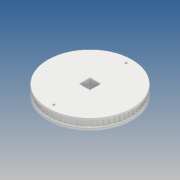
# Autodesk Inventor part: Poleas de transmision 60Dientes (ZR timing belts)
Saved by Autodesk Inventor 2020 (Build 240168000, 168)
## iProperties
Part Number: Poleas de transmision 60Dientes (ZR timing belts)
Material: Genérico
Document SubType Name: Modeling
Designer: FABLAB
Density: 1 g/cm^3
Appearance: Blanco
Description: Acrílico corte laser CNC
Author: FABLAB
Autodesk Inventor part; units mm, degrees
ref_plane "YZ Plane" through (0, 0, 0) normal (1, 0, 0) x (0, 1, 0)
ref_plane "XZ Plane" through (0, 0, 0) normal (0, 1, 0) x (-1, 0, 0)
ref_plane "XY Plane" through (0, 0, 0) normal (0, 0, 1) x (1, 0, 0)
sketch "Boceto1" plane through (0, 0, 0) normal (0, 0, 1) x (1, 0, 0)
  line L0 (8, -8) -> (-8, -8) projected
  line L1 (-8, -8) -> (-8, 8) projected
  line L2 (-8, 8) -> (8, 8) projected
  line L3 (8, 8) -> (8, -8) projected
  circle A0 centre (0, 0) radius 15 construction
  circle A1 centre (0, 0) radius 60
  circle A2 centre (0, 0) radius 55 construction
  circle A3 centre (0, 55) radius 1.5
  circle A4 centre (0, -55) radius 1.5
  circle A5 centre (0, 0) radius 61.2874 construction
  line L4 (-1.5392, 59.9803) -> (1.5392, 59.9803)
  line L5 (1.5392, 59.9803) -> (0.933, 61.2803)
  line L6 (0.933, 61.2803) -> (-0.933, 61.2803)
  line L7 (-0.933, 61.2803) -> (-1.5392, 59.9803)
  line L8 (0, 59.9803) -> (0, 0) construction
  line L9 (0, 0) -> (2.5392, 59.9462) construction
  line L10 (0, 0) -> (-2.5392, 59.9462) construction
  arc A6 (-2.5392, 59.9462) -> (2.5392, 59.9462) centre (0, 119.8925) ccw construction
  line L11 (1.5392, 59.9803) -> (1.5392, 62.0856) construction
  line L12 (-7.3335, 60.847) -> (-7.8005, 59.4908)
  line L13 (-5.4776, 61.0421) -> (-7.3335, 60.847)
  line L14 (-4.7388, 59.8126) -> (-5.4776, 61.0421)
  line L15 (-13.6535, 59.7471) -> (-13.9762, 58.3495)
  line L16 (-11.8282, 60.1351) -> (-13.6535, 59.7471)
  line L17 (-10.965, 58.9896) -> (-11.8282, 60.1351)
  line L18 (-19.824, 57.9927) -> (-19.9988, 56.569)
  line L19 (-18.0493, 58.5693) -> (-19.824, 57.9927)
  line L20 (-17.071, 57.5203) -> (-18.0493, 58.5693)
  line L21 (-25.7773, 55.6028) -> (-25.8023, 54.1686)
  line L22 (-24.0725, 56.3618) -> (-25.7773, 55.6028)
  line L23 (-22.99, 55.4208) -> (-24.0725, 56.3618)
  line L24 (-31.4482, 52.6037) -> (-31.3231, 51.1748)
  line L25 (-29.8321, 53.5368) -> (-31.4482, 52.6037)
  line L26 (-28.6571, 52.714) -> (-29.8321, 53.5368)
  line L27 (-36.7745, 49.0283) -> (-36.5008, 47.6203)
  line L28 (-35.2648, 50.1252) -> (-36.7745, 49.0283)
  line L29 (-34.0102, 49.4298) -> (-35.2648, 50.1252)
  line L30 (-41.6979, 44.9158) -> (-41.2785, 43.5441)
  line L31 (-40.3111, 46.1644) -> (-41.6979, 44.9158)
  line L32 (-38.9907, 45.604) -> (-40.3111, 46.1644)
  line L33 (-46.1644, 40.3111) -> (-45.604, 38.9907)
  line L34 (-44.9158, 41.6979) -> (-46.1644, 40.3111)
  line L35 (-43.5441, 41.2785) -> (-44.9158, 41.6979)
  line L36 (-50.1252, 35.2648) -> (-49.4298, 34.0102)
  line L37 (-49.0283, 36.7745) -> (-50.1252, 35.2648)
  line L38 (-47.6203, 36.5008) -> (-49.0283, 36.7745)
  line L39 (-53.5368, 29.8321) -> (-52.714, 28.6571)
  line L40 (-52.6037, 31.4482) -> (-53.5368, 29.8321)
  line L41 (-51.1748, 31.3231) -> (-52.6037, 31.4482)
  line L42 (-56.3618, 24.0725) -> (-55.4208, 22.99)
  line L43 (-55.6028, 25.7773) -> (-56.3618, 24.0725)
  line L44 (-54.1686, 25.8023) -> (-55.6028, 25.7773)
  line L45 (-58.5693, 18.0493) -> (-57.5203, 17.071)
  line L46 (-57.9927, 19.824) -> (-58.5693, 18.0493)
  line L47 (-56.569, 19.9988) -> (-57.9927, 19.824)
  line L48 (-60.1351, 11.8282) -> (-58.9896, 10.965)
  line L49 (-59.7471, 13.6535) -> (-60.1351, 11.8282)
  line L50 (-58.3495, 13.9762) -> (-59.7471, 13.6535)
  line L51 (-61.0421, 5.4776) -> (-59.8126, 4.7388)
  line L52 (-60.847, 7.3335) -> (-61.0421, 5.4776)
  line L53 (-59.4908, 7.8005) -> (-60.847, 7.3335)
  line L54 (-61.2803, -0.933) -> (-59.9803, -1.5392)
  line L55 (-61.2803, 0.933) -> (-61.2803, -0.933)
  line L56 (-59.9803, 1.5392) -> (-61.2803, 0.933)
  line L57 (-60.847, -7.3335) -> (-59.4908, -7.8005)
  line L58 (-61.0421, -5.4776) -> (-60.847, -7.3335)
  line L59 (-59.8126, -4.7388) -> (-61.0421, -5.4776)
  line L60 (-59.7471, -13.6535) -> (-58.3495, -13.9762)
  line L61 (-60.1351, -11.8282) -> (-59.7471, -13.6535)
  line L62 (-58.9896, -10.965) -> (-60.1351, -11.8282)
  line L63 (-57.9927, -19.824) -> (-56.569, -19.9988)
  line L64 (-58.5693, -18.0493) -> (-57.9927, -19.824)
  line L65 (-57.5203, -17.071) -> (-58.5693, -18.0493)
  line L66 (-55.6028, -25.7773) -> (-54.1686, -25.8023)
  line L67 (-56.3618, -24.0725) -> (-55.6028, -25.7773)
  line L68 (-55.4208, -22.99) -> (-56.3618, -24.0725)
  line L69 (-52.6037, -31.4482) -> (-51.1748, -31.3231)
  line L70 (-53.5368, -29.8321) -> (-52.6037, -31.4482)
  line L71 (-52.714, -28.6571) -> (-53.5368, -29.8321)
  line L72 (-49.0283, -36.7745) -> (-47.6203, -36.5008)
  line L73 (-50.1252, -35.2648) -> (-49.0283, -36.7745)
  line L74 (-49.4298, -34.0102) -> (-50.1252, -35.2648)
  line L75 (-44.9158, -41.6979) -> (-43.5441, -41.2785)
  line L76 (-46.1644, -40.3111) -> (-44.9158, -41.6979)
  line L77 (-45.604, -38.9907) -> (-46.1644, -40.3111)
  line L78 (-40.3111, -46.1644) -> (-38.9907, -45.604)
  line L79 (-41.6979, -44.9158) -> (-40.3111, -46.1644)
  line L80 (-41.2785, -43.5441) -> (-41.6979, -44.9158)
  line L81 (-35.2648, -50.1252) -> (-34.0102, -49.4298)
  line L82 (-36.7745, -49.0283) -> (-35.2648, -50.1252)
  line L83 (-36.5008, -47.6203) -> (-36.7745, -49.0283)
  line L84 (-29.8321, -53.5368) -> (-28.6571, -52.714)
  line L85 (-31.4482, -52.6037) -> (-29.8321, -53.5368)
  line L86 (-31.3231, -51.1748) -> (-31.4482, -52.6037)
  line L87 (-24.0725, -56.3618) -> (-22.99, -55.4208)
  line L88 (-25.7773, -55.6028) -> (-24.0725, -56.3618)
  line L89 (-25.8023, -54.1686) -> (-25.7773, -55.6028)
  line L90 (-18.0493, -58.5693) -> (-17.071, -57.5203)
  line L91 (-19.824, -57.9927) -> (-18.0493, -58.5693)
  line L92 (-19.9988, -56.569) -> (-19.824, -57.9927)
  line L93 (-11.8282, -60.1351) -> (-10.965, -58.9896)
  line L94 (-13.6535, -59.7471) -> (-11.8282, -60.1351)
  line L95 (-13.9762, -58.3495) -> (-13.6535, -59.7471)
  line L96 (-5.4776, -61.0421) -> (-4.7388, -59.8126)
  line L97 (-7.3335, -60.847) -> (-5.4776, -61.0421)
  line L98 (-7.8005, -59.4908) -> (-7.3335, -60.847)
  line L99 (0.933, -61.2803) -> (1.5392, -59.9803)
  line L100 (-0.933, -61.2803) -> (0.933, -61.2803)
  line L101 (-1.5392, -59.9803) -> (-0.933, -61.2803)
  line L102 (7.3335, -60.847) -> (7.8005, -59.4908)
  line L103 (5.4776, -61.0421) -> (7.3335, -60.847)
  line L104 (4.7388, -59.8126) -> (5.4776, -61.0421)
  line L105 (13.6535, -59.7471) -> (13.9762, -58.3495)
  line L106 (11.8282, -60.1351) -> (13.6535, -59.7471)
  line L107 (10.965, -58.9896) -> (11.8282, -60.1351)
  line L108 (19.824, -57.9927) -> (19.9988, -56.569)
  line L109 (18.0493, -58.5693) -> (19.824, -57.9927)
  line L110 (17.071, -57.5203) -> (18.0493, -58.5693)
  line L111 (25.7773, -55.6028) -> (25.8023, -54.1686)
  line L112 (24.0725, -56.3618) -> (25.7773, -55.6028)
  line L113 (22.99, -55.4208) -> (24.0725, -56.3618)
  line L114 (31.4482, -52.6037) -> (31.3231, -51.1748)
  line L115 (29.8321, -53.5368) -> (31.4482, -52.6037)
  line L116 (28.6571, -52.714) -> (29.8321, -53.5368)
  line L117 (36.7745, -49.0283) -> (36.5008, -47.6203)
  line L118 (35.2648, -50.1252) -> (36.7745, -49.0283)
  line L119 (34.0102, -49.4298) -> (35.2648, -50.1252)
  line L120 (41.6979, -44.9158) -> (41.2785, -43.5441)
  line L121 (40.3111, -46.1644) -> (41.6979, -44.9158)
  line L122 (38.9907, -45.604) -> (40.3111, -46.1644)
  line L123 (46.1644, -40.3111) -> (45.604, -38.9907)
  line L124 (44.9158, -41.6979) -> (46.1644, -40.3111)
  line L125 (43.5441, -41.2785) -> (44.9158, -41.6979)
  line L126 (50.1252, -35.2648) -> (49.4298, -34.0102)
  line L127 (49.0283, -36.7745) -> (50.1252, -35.2648)
  line L128 (47.6203, -36.5008) -> (49.0283, -36.7745)
  line L129 (53.5368, -29.8321) -> (52.714, -28.6571)
  line L130 (52.6037, -31.4482) -> (53.5368, -29.8321)
  line L131 (51.1748, -31.3231) -> (52.6037, -31.4482)
  line L132 (56.3618, -24.0725) -> (55.4208, -22.99)
  line L133 (55.6028, -25.7773) -> (56.3618, -24.0725)
  line L134 (54.1686, -25.8023) -> (55.6028, -25.7773)
  line L135 (58.5693, -18.0493) -> (57.5203, -17.071)
  line L136 (57.9927, -19.824) -> (58.5693, -18.0493)
  line L137 (56.569, -19.9988) -> (57.9927, -19.824)
  line L138 (60.1351, -11.8282) -> (58.9896, -10.965)
  line L139 (59.7471, -13.6535) -> (60.1351, -11.8282)
  line L140 (58.3495, -13.9762) -> (59.7471, -13.6535)
  line L141 (61.0421, -5.4776) -> (59.8126, -4.7388)
  line L142 (60.847, -7.3335) -> (61.0421, -5.4776)
  line L143 (59.4908, -7.8005) -> (60.847, -7.3335)
  line L144 (61.2803, 0.933) -> (59.9803, 1.5392)
  line L145 (61.2803, -0.933) -> (61.2803, 0.933)
  line L146 (59.9803, -1.5392) -> (61.2803, -0.933)
  line L147 (60.847, 7.3335) -> (59.4908, 7.8005)
  line L148 (61.0421, 5.4776) -> (60.847, 7.3335)
  line L149 (59.8126, 4.7388) -> (61.0421, 5.4776)
  line L150 (59.7471, 13.6535) -> (58.3495, 13.9762)
  line L151 (60.1351, 11.8282) -> (59.7471, 13.6535)
  line L152 (58.9896, 10.965) -> (60.1351, 11.8282)
  line L153 (57.9927, 19.824) -> (56.569, 19.9988)
  line L154 (58.5693, 18.0493) -> (57.9927, 19.824)
  line L155 (57.5203, 17.071) -> (58.5693, 18.0493)
  line L156 (55.6028, 25.7773) -> (54.1686, 25.8023)
  line L157 (56.3618, 24.0725) -> (55.6028, 25.7773)
  line L158 (55.4208, 22.99) -> (56.3618, 24.0725)
  line L159 (52.6037, 31.4482) -> (51.1748, 31.3231)
  line L160 (53.5368, 29.8321) -> (52.6037, 31.4482)
  line L161 (52.714, 28.6571) -> (53.5368, 29.8321)
  line L162 (49.0283, 36.7745) -> (47.6203, 36.5008)
  line L163 (50.1252, 35.2648) -> (49.0283, 36.7745)
  line L164 (49.4298, 34.0102) -> (50.1252, 35.2648)
  line L165 (44.9158, 41.6979) -> (43.5441, 41.2785)
  line L166 (46.1644, 40.3111) -> (44.9158, 41.6979)
  line L167 (45.604, 38.9907) -> (46.1644, 40.3111)
  line L168 (40.3111, 46.1644) -> (38.9907, 45.604)
  line L169 (41.6979, 44.9158) -> (40.3111, 46.1644)
  line L170 (41.2785, 43.5441) -> (41.6979, 44.9158)
  line L171 (35.2648, 50.1252) -> (34.0102, 49.4298)
  line L172 (36.7745, 49.0283) -> (35.2648, 50.1252)
  line L173 (36.5008, 47.6203) -> (36.7745, 49.0283)
  line L174 (29.8321, 53.5368) -> (28.6571, 52.714)
  line L175 (31.4482, 52.6037) -> (29.8321, 53.5368)
  line L176 (31.3231, 51.1748) -> (31.4482, 52.6037)
  line L177 (24.0725, 56.3618) -> (22.99, 55.4208)
  line L178 (25.7773, 55.6028) -> (24.0725, 56.3618)
  line L179 (25.8023, 54.1686) -> (25.7773, 55.6028)
  line L180 (18.0493, 58.5693) -> (17.071, 57.5203)
  line L181 (19.824, 57.9927) -> (18.0493, 58.5693)
  line L182 (19.9988, 56.569) -> (19.824, 57.9927)
  line L183 (11.8282, 60.1351) -> (10.965, 58.9896)
  line L184 (13.6535, 59.7471) -> (11.8282, 60.1351)
  line L185 (13.9762, 58.3495) -> (13.6535, 59.7471)
  line L186 (5.4776, 61.0421) -> (4.7388, 59.8126)
  line L187 (7.3335, 60.847) -> (5.4776, 61.0421)
  line L188 (7.8005, 59.4908) -> (7.3335, 60.847)
  point P0 (0, 61.2803)
  point P1 (-6.4055, 60.9446)
  point P2 (-12.7409, 59.9411)
  point P3 (-18.9366, 58.281)
  point P4 (-24.9249, 55.9823)
  point P5 (-30.6401, 53.0703)
  point P6 (-36.0196, 49.5768)
  point P7 (-41.0045, 45.5401)
  point P8 (-45.5401, 41.0045)
  point P9 (-49.5768, 36.0196)
  point P10 (-53.0703, 30.6401)
  point P11 (-55.9823, 24.9249)
  point P12 (-58.281, 18.9366)
  point P13 (-59.9411, 12.7409)
  point P14 (-60.9446, 6.4055)
  point P15 (-61.2803, 0)
  point P16 (-60.9446, -6.4055)
  point P17 (-59.9411, -12.7409)
  point P18 (-58.281, -18.9366)
  point P19 (-55.9823, -24.9249)
  point P20 (-53.0703, -30.6401)
  point P21 (-49.5768, -36.0196)
  point P22 (-45.5401, -41.0045)
  point P23 (-41.0045, -45.5401)
  point P24 (-36.0196, -49.5768)
  point P25 (-30.6401, -53.0703)
  point P26 (-24.9249, -55.9823)
  point P27 (-18.9366, -58.281)
  point P28 (-12.7409, -59.9411)
  point P29 (-6.4055, -60.9446)
  point P30 (-38.9907, -45.604)
  point P31 (-36.5008, -47.6203)
  point P32 (-31.3231, -51.1748)
  point P33 (-28.6571, -52.714)
  point P34 (-25.8023, -54.1686)
  point P35 (-22.99, -55.4208)
  point P36 (-19.9988, -56.569)
  point P37 (-17.071, -57.5203)
  point P38 (-13.9762, -58.3495)
  point P39 (-10.965, -58.9896)
  point P40 (-7.8005, -59.4908)
  point P41 (-4.7388, -59.8126)
  point P42 (-1.5392, 59.9803)
  point P43 (-4.7388, 59.8126)
  point P44 (-7.8005, 59.4908)
  point P45 (-10.965, 58.9896)
  point P46 (-13.9762, 58.3495)
  point P47 (-17.071, 57.5203)
  point P48 (-19.9988, 56.569)
  point P49 (-22.99, 55.4208)
  point P50 (-25.8023, 54.1686)
  point P51 (-28.6571, 52.714)
  point P52 (-31.3231, 51.1748)
  point P53 (-34.0102, 49.4298)
  point P54 (-36.5008, 47.6203)
  point P55 (-38.9907, 45.604)
  point P56 (-43.5441, 41.2785)
  point P57 (-45.604, 38.9907)
  point P58 (-47.6203, 36.5008)
  point P59 (-49.4298, 34.0102)
  point P60 (-51.1748, 31.3231)
  point P61 (-54.1686, 25.8023)
  point P62 (-55.4208, 22.99)
  point P63 (-56.569, 19.9988)
  point P64 (-57.5203, 17.071)
  point P65 (-58.3495, 13.9762)
  point P66 (-58.9896, 10.965)
  point P67 (-59.4908, 7.8005)
  point P68 (-59.8126, 4.7388)
  point P69 (-59.9803, 1.5392)
  point P70 (-59.9803, -1.5392)
  point P71 (-59.8126, -4.7388)
  point P72 (-59.4908, -7.8005)
  point P73 (-58.9896, -10.965)
  point P74 (-58.3495, -13.9762)
  point P75 (-57.5203, -17.071)
  point P76 (-56.569, -19.9988)
  point P77 (-55.4208, -22.99)
  point P78 (-52.714, -28.6571)
  point P79 (-51.1748, -31.3231)
  point P80 (-49.4298, -34.0102)
  point P81 (-47.6203, -36.5008)
  point P82 (-45.604, -38.9907)
  point P83 (-43.5441, -41.2785)
  point P84 (-41.2785, -43.5441)
  point P85 (0, -61.2803)
  point P86 (6.4055, -60.9446)
  point P87 (12.7409, -59.9411)
  point P88 (18.9366, -58.281)
  point P89 (24.9249, -55.9823)
  point P90 (30.6401, -53.0703)
  point P91 (36.0196, -49.5768)
  point P92 (41.0045, -45.5401)
  point P93 (45.5401, -41.0045)
  point P94 (49.5768, -36.0196)
  point P95 (53.0703, -30.6401)
  point P96 (55.9823, -24.9249)
  point P97 (58.281, -18.9366)
  point P98 (59.9411, -12.7409)
  point P99 (60.9446, -6.4055)
  point P100 (61.2803, 0)
  point P101 (60.9446, 6.4055)
  point P102 (59.9411, 12.7409)
  point P103 (58.281, 18.9366)
  point P104 (55.9823, 24.9249)
  point P105 (53.0703, 30.6401)
  point P106 (49.5768, 36.0196)
  point P107 (45.5401, 41.0045)
  point P108 (41.0045, 45.5401)
  point P109 (36.0196, 49.5768)
  point P110 (30.6401, 53.0703)
  point P111 (24.9249, 55.9823)
  point P112 (18.9366, 58.281)
  point P113 (12.7409, 59.9411)
  point P114 (6.4055, 60.9446)
  dimension "d4" = 5
  dimension "d24" = 122.5747
  dimension "diametro" = 120
  dimension "d3" = 3
  dimension "d7" = 360
  dimension "d25" = 1.3
  dimension "d26" = 5.0785
  dimension "diente" = 5.08
  dimension "d28" = 25
  dimension "d29" = 50
  dimension "d30" = 3.0785
  dimension "d33" = 360
  constraints: 370 end point, 4 vertical alignment, 3 centre point, 3 coincident, 2 midpoint, 2 point on circle, 2 vertical, 1 equal length, 1 horizontal, 1 parallel, 497 other
  measures "d3" diameter of A3
  measures "d25" vertical distance of L4.end L5.end
  measures "d26" distance of L9.end L10.end
  measures "d28" angle of L8 L5
  measures "d29" angle of L5 L7
  measures "d30" distance of L4.end L4.start
extrude "Extrusión1" add sketch "Boceto1" along normal blind 10
sketch "Boceto2" plane through (0, 0, 0) normal (0, 0, -1) x (-1, 0, 0)
  circle A0 centre (0, 0) radius 64
  circle A1 centre (0, 0) radius 46
  circle A2 centre (0, 55) radius 1.5 projected
  circle A3 centre (0, -55) radius 1.5 projected
  circle A4 centre (0, -55) radius 1.5 construction
  circle A5 centre (0, -55) radius 9 construction
  dimension "d9" = 92
  dimension "d21" = 128
  constraints: 4 coincident, 3 centre point, 2 tangent
  measures "d9" diameter of A1
  measures "d21" diameter of A0
extrude "Extrusión2" add sketch "Boceto2" along normal blind 3 separate body
sketch "Boceto3" plane through (0, 0, 10) normal (0, 0, 1) x (1, 0, 0)
  circle A0 centre (0, 0) radius 64 projected
  circle A1 centre (0, 55) radius 1.5 projected
  circle A2 centre (0, -55) radius 1.5 projected
  line L0 (8, 8) -> (-8, 8) projected
  line L1 (8, -8) -> (8, 8) projected
  line L2 (-8, -8) -> (8, -8) projected
  line L3 (-8, 8) -> (-8, -8) projected
extrude "Extrusión3" add sketch "Boceto3" along normal blind 3 separate body
equation "\"diametro\" = 2 * dientes"
equation "\"dientes\" = 60"
